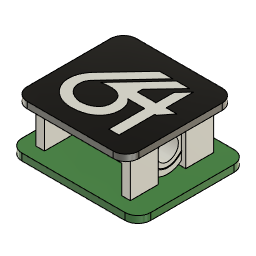
C64_logo_illuminated_multi v5 (Autodesk Fusion 360 design; units mm, degrees)
Autodesk Fusion 360 part; units mm, degrees
sketch "face plate" plane through (0, 0, 0) normal (0, 0, 1) x (1, 0, 0) in component "Face Plate"
  arc A0 (13, 9.7) -> (10, 12.7) centre (10, 9.7) ccw
  arc A1 (-13, -9.7) -> (-10, -12.7) centre (-10, -9.7) ccw
  arc A2 (10, -12.7) -> (13, -9.7) centre (10, -9.7) ccw
  line L0 (-13, 12.7) -> (13, -12.7) construction
  line L1 (-10, -12.7) -> (10, -12.7)
  arc A3 (-10, 12.7) -> (-13, 9.7) centre (-10, 9.7) ccw
  line L2 (10, 12.7) -> (-10, 12.7)
  line L3 (13, -9.7) -> (13, 9.7)
  line L4 (-10, 9.7) -> (10, -9.7) construction
  line L5 (13, 12.7) -> (-13, -12.7) construction
  line L6 (-10, -9.7) -> (10, -9.7) construction
  line L7 (10, 9.7) -> (-10, -9.7) construction
  line L8 (10, 9.7) -> (-10, 9.7) construction
  line L9 (-13, 9.7) -> (-13, -9.7)
  line L10 (10, -9.7) -> (10, 9.7) construction
  line L11 (-10, 9.7) -> (-10, -9.7) construction
  spline S0 degree 3 poles (2.5906, -3.5962) (2.5376, -1.7674) (1.7387, -0.8132) (1.1259, -0.4461) knots 0 0 0 0 1 1 1 1
  line L12 (2.5906, -3.5962) -> (2.5376, -1.7674)
  line L13 (2.5376, -1.7674) -> (1.7387, -0.8132)
  line L14 (1.7387, -0.8132) -> (1.1259, -0.4461)
  spline S1 degree 3 poles (-9.888, -3.2279) (-9.888, -6.2686) (-7.0983, -8.7953) (-3.8691, -8.7953) knots 0 0 0 0 1 1 1 1
  line L15 (-9.888, -3.2279) -> (-9.888, -6.2686)
  line L16 (-9.888, -6.2686) -> (-7.0983, -8.7953)
  line L17 (-7.0983, -8.7953) -> (-3.8691, -8.7953)
  line L18 (7.4492, -8.7953) -> (7.4492, -0.4461)
  line L19 (7.4492, -0.4461) -> (7.8267, -0.4474)
  spline S2 degree 3 poles (-3.8691, -8.7953) (0.9243, -8.7953) (2.6578, -5.9391) (2.5906, -3.5962) knots 0 0 0 0 1 1 1 1
  line L20 (-3.8691, -8.7953) -> (0.9243, -8.7953)
  line L21 (0.9243, -8.7953) -> (2.6578, -5.9391)
  line L22 (2.6578, -5.9391) -> (2.5906, -3.5962)
  spline S3 degree 3 poles (-3.8684, -6.5605) (-4.8205, -6.5605) (-7.4292, -5.7507) (-7.5798, -3.3049) knots 0 0 0 0 1 1 1 1
  line L23 (-3.8684, -6.5605) -> (-4.8205, -6.5605)
  line L24 (-4.8205, -6.5605) -> (-7.4292, -5.7507)
  line L25 (-7.4292, -5.7507) -> (-7.5798, -3.3049)
  line L26 (5.0693, -0.4461) -> (5.0693, -8.7953)
  line L27 (5.0693, -8.7953) -> (7.4492, -8.7953)
  spline S4 degree 2 poles (-7.5798, -3.3049) (-7.6755, -1.7654) (-6.5786, -0.7329) knots 0 0 0 1 1 1
  line L28 (-7.5798, -3.3049) -> (-7.6755, -1.7654)
  line L29 (-7.6755, -1.7654) -> (-6.5786, -0.7329)
  spline S5 degree 3 poles (0.1739, -3.0822) (0.2818, -5.6121) (-1.9966, -6.5605) (-3.8684, -6.5605) knots 0 0 0 0 1 1 1 1
  line L30 (0.1739, -3.0822) -> (0.2818, -5.6121)
  line L31 (0.2818, -5.6121) -> (-1.9966, -6.5605)
  line L32 (-1.9966, -6.5605) -> (-3.8684, -6.5605)
  line L33 (7.8267, -0.4474) -> (9.9138, 2.2094)
  spline S6 degree 2 poles (-5.295, -0.3005) (0.0123, 0.7243) (0.1739, -3.0822) knots 0 0 0 1 1 1
  line L34 (-5.295, -0.3005) -> (0.0123, 0.7243)
  line L35 (0.0123, 0.7243) -> (0.1739, -3.0822)
  line L36 (5.2394, 2.0437) -> (0.9553, 2.0437)
  spline S7 degree 2 poles (-8.3212, 0.7243) (-9.888, -1.1323) (-9.888, -3.2279) knots 0 0 0 1 1 1
  line L37 (-8.3212, 0.7243) -> (-9.888, -1.1323)
  line L38 (-9.888, -1.1323) -> (-9.888, -3.2279)
  line L39 (-0.6729, 8.8158) -> (-8.3212, 0.7243)
  line L40 (0.9553, 3.1785) -> (6.2962, 8.8158)
  line L41 (7.4493, 8.5608) -> (5.2394, 6.181)
  line L42 (-6.5786, -0.7329) -> (2.3527, 8.8159)
  line L43 (5.2394, 6.181) -> (5.2394, 2.0437)
  line L44 (7.4493, 2.2094) -> (7.4493, 8.5608)
  line L45 (6.2962, 8.8158) -> (3.237, 8.8158)
  line L46 (2.3527, 8.8159) -> (-0.6729, 8.8158)
  line L47 (1.1259, -0.4461) -> (5.0693, -0.4461)
  line L48 (3.237, 8.8158) -> (-5.295, -0.3005)
  line L49 (0.9553, 2.0437) -> (0.9553, 3.1785)
  line L50 (9.9138, 2.2094) -> (7.4493, 2.2094)
  dimension "d101" = 20
  dimension "d102" = 19.4
  dimension "d103" = 3
  dimension "d104" = 3
  dimension "d105" = 3
  dimension "d106" = 3
  dimension "d107" = 3
  dimension "d108" = 3
  constraint perpendicular L8 L11
  constraint parallel L6 L8
  constraint horizontal L8
  constraint parallel L1 L2
  constraint horizontal L2
  constraint coincident L5.end L9
  constraint coincident L5.end L1
  constraint tangent A1 L9
  constraint tangent A1 L1
  constraint coincident L0.end L1
  constraint coincident L0.end L3
  constraint tangent A2 L1
  constraint tangent A2 L3
  constraint coincident L5.start L2
  constraint coincident L5.start L3
  constraint tangent A0 L2
  constraint tangent A0 L3
  constraint coincident L0.start L9
  constraint coincident L0.start L2
  constraint tangent A3 L9
  constraint tangent A3 L2
  measures "d101" distance of A1.centre A2.centre
  measures "d102" distance of A3.centre A1.centre
  measures "d103" distance of L9 L11
  measures "d104" distance of L1 L6
  measures "d105" radius of A1
  measures "d106" radius of A2
  measures "d107" radius of A0
  measures "d108" radius of A3
sketch "illuminated body" plane through (0, 0, 0) normal (0, 0, 1) x (1, 0, 0) in component "Illuminated_Body_multi"
  line L0 (-10, 9.7) -> (-10, -9.7)
  line L1 (10, 9.7) -> (-10, 9.7)
  line L2 (10, -9.7) -> (10, 9.7)
  line L3 (-10, -9.7) -> (10, -9.7)
  spline S0 degree 3 poles (-9.888, -3.2279) (-9.888, -6.2686) (-7.0983, -8.7953) (-3.8691, -8.7953) knots 0 0 0 0 1 1 1 1
  spline S1 degree 2 poles (-8.3212, 0.7243) (-9.888, -1.1323) (-9.888, -3.2279) knots 0 0 0 1 1 1
  line L4 (-0.6729, 8.8158) -> (-8.3212, 0.7243)
  line L5 (2.3527, 8.8159) -> (-0.6729, 8.8158)
  line L6 (-6.5786, -0.7329) -> (2.3527, 8.8159)
  spline S2 degree 2 poles (-7.5798, -3.3049) (-7.6755, -1.7654) (-6.5786, -0.7329) knots 0 0 0 1 1 1
  spline S3 degree 3 poles (-3.8684, -6.5605) (-4.8205, -6.5605) (-7.4292, -5.7507) (-7.5798, -3.3049) knots 0 0 0 0 1 1 1 1
  spline S4 degree 3 poles (0.1739, -3.0822) (0.2818, -5.6121) (-1.9966, -6.5605) (-3.8684, -6.5605) knots 0 0 0 0 1 1 1 1
  spline S5 degree 2 poles (-5.295, -0.3005) (0.0123, 0.7243) (0.1739, -3.0822) knots 0 0 0 1 1 1
  line L7 (3.237, 8.8158) -> (-5.295, -0.3005)
  line L8 (6.2962, 8.8158) -> (3.237, 8.8158)
  line L9 (0.9553, 3.1785) -> (6.2962, 8.8158)
  line L10 (0.9553, 2.0437) -> (0.9553, 3.1785)
  line L11 (5.2394, 2.0437) -> (0.9553, 2.0437)
  line L12 (5.2394, 6.181) -> (5.2394, 2.0437)
  line L13 (7.4493, 8.5608) -> (5.2394, 6.181)
  line L14 (7.4493, 2.2094) -> (7.4493, 8.5608)
  line L15 (9.9138, 2.2094) -> (7.4493, 2.2094)
  line L16 (7.8267, -0.4474) -> (9.9138, 2.2094)
  line L17 (7.4492, -0.4461) -> (7.8267, -0.4474)
  line L18 (7.4492, -8.7953) -> (7.4492, -0.4461)
  line L19 (5.0693, -8.7953) -> (7.4492, -8.7953)
  line L20 (5.0693, -0.4461) -> (5.0693, -8.7953)
  line L21 (1.1259, -0.4461) -> (5.0693, -0.4461)
  spline S6 degree 3 poles (2.5906, -3.5962) (2.5376, -1.7674) (1.7387, -0.8132) (1.1259, -0.4461) knots 0 0 0 0 1 1 1 1
  spline S7 degree 3 poles (-3.8691, -8.7953) (0.9243, -8.7953) (2.6578, -5.9391) (2.5906, -3.5962) knots 0 0 0 0 1 1 1 1
extrude "Extrude1" add sketch "illuminated body" against normal blind 1 contours L0 L1 L2 L3 | S0 S1 L4 L5 L6 S2 S3 S4 S5 L7 L8 L9 L10 L11 L12 L13 L14 L15 L16 L17 L18 L19 L20 L21 S6 S7 makes body 1 in component "Illuminated_Body_multi"
extrude "Extrude2" add sketch "face plate" along normal blind 1.5 contours S0 S1 L18 L19 S2 L23 L24 L25 L26 L27 L28 L29 L30 L31 L32 L33 L34 L35 L36 S7 L39 L40 L41 L42 L43 L44 L45 L46 L47 L48 L49 L50 | S4 L28 L29 | S3 L23 L24 L25 | S5 L30 L31 L32 | S6 L34 L35 bodies 1 in component "Illuminated_Body_multi"
extrude "Extrude1'" add sketch "face plate" along normal blind 1.5 separate body contours A0 A1 A2 L1 A3 L2 L3 L9 | S0 L12 L13 L14 | S2 L20 L21 L22 | S1 L15 L16 L17 | S7 L37 L38 makes body 2 in component "Face Plate"
sketch "led insert" plane through (10, 0, 0) normal (1, 0, 0) x (0, 1, 0) in component "Illuminated_Body_multi"
  line L0 (9.7, 0) -> (-9.7, 0)
  line L1 (-9.7, 0) -> (-9.7, -1)
  line L2 (-9.7, -1) -> (9.7, -1)
  line L3 (9.7, -1) -> (9.7, 0)
  line L4 (0, -1) -> (0, -9.1868) construction
  line L5 (-9.7, -1) -> (-2.2348, -7.1936)
  line L6 (-9.7, -1) -> (9.7, -1)
  line L7 (9.7, -1) -> (2.2348, -7.1936)
  circle A0 centre (0, -4.5) radius 2.5
  line L8 (9.7, -1) -> (-9.7, -1)
  arc A1 (-2.2348, -7.1936) -> (2.2348, -7.1936) centre (0, -4.5) ccw
  dimension "d115" = 5
  dimension "d116" = 3.5
  dimension "d117" = 7
  constraint midpoint L4.start L6
  constraint coincident A0.centre L4
  constraint concentric A0 A1
  constraint coincident L1.end L2.start
  constraint tangent L5 A1
  constraint coincident L2.end L3.start
  constraint tangent L7 A1
  measures "d115" diameter of A0
  measures "d116" distance of A0.centre L8
  measures "d117" diameter of A1
extrude "Extrude3" add sketch "led insert" against normal blind 20 contours L2 L5 L6 L7 L8 A1 bodies 1 in component "Illuminated_Body_multi"
sketch "reflector" plane through (10, 0, 0) normal (1, 0, 0) x (0, 1, 0) in component "Refector"
  circle A0 centre (0, -4.5) radius 2.5
  line L0 (9.7, 0) -> (-9.7, 0)
  line L1 (-9.7, 0) -> (-9.7, -1)
  line L2 (-9.7, -1) -> (-2.2348, -7.1936)
  arc A1 (-2.2348, -7.1936) -> (2.2348, -7.1936) centre (0, -4.5) ccw
  line L3 (2.2348, -7.1936) -> (9.7, -1)
  line L4 (9.7, -1) -> (9.7, 0)
  line L5 (-9.7, -2.949) -> (-9.7, -9.5)
  line L6 (-3.2, -9.5) -> (-9.7, -9.5)
  line L7 (9.7, -1) -> (9.7, 0)
  line L8 (9.7, -1.2599) -> (9.7, -2.949)
  arc A2 (-3.1926, -8.348) -> (3.1926, -8.348) centre (0, -4.5) ccw
  line L9 (0, -9.5) -> (9.7, -9.5)
  arc A3 (-2.3625, -7.3475) -> (2.3625, -7.3475) centre (0, -4.5) ccw
  line L10 (9.7, -1.2599) -> (3.2, -1.2599)
  line L11 (3.1926, -8.348) -> (9.7, -2.949)
  line L12 (9.7, -9.5) -> (9.7, -2.949)
  line L13 (-9.7, 0) -> (-9.7, -1)
  line L14 (-9.7, -1.2599) -> (-9.7, -2.949)
  line L15 (3.2, -9.5) -> (9.7, -9.5)
  line L16 (-9.7, -1.2599) -> (-2.3625, -7.3475)
  line L17 (-9.7, -9.5) -> (0, -9.5)
  circle A4 centre (0, -4.5) radius 2.5
  line L18 (-3.2, -1.2599) -> (-3.2, -9.5)
  line L19 (-9.7, -2.949) -> (-3.1926, -8.348)
  line L20 (-9.7, -9.5) -> (-9.7, -1.2599)
  line L21 (-9.7, -1.2599) -> (-3.2, -1.2599)
  line L22 (3.2, -1.2599) -> (3.2, -9.5)
  line L23 (2.3625, -7.3475) -> (9.7, -1.2599)
  line L24 (9.7, 0) -> (-9.7, 0)
  line L25 (9.7, -9.5) -> (9.7, -1.2599)
  line L26 (-9.7, -1) -> (-2.2348, -7.1936) construction
  arc A5 (-2.2348, -7.1936) -> (2.2348, -7.1936) centre (0, -4.5) ccw construction
  line L27 (9.7, -1) -> (2.2348, -7.1936) construction
  line L28 (9.7, -1) -> (9.7, 0) construction
  line L29 (-9.7, 0) -> (9.7, 0) construction
  line L30 (-9.7, 0) -> (-9.7, -1) construction
  dimension "d121" = 1.3
  dimension "d122" = 9.7
  dimension "d123" = 19.4
  dimension "d124" = 6.5
  dimension "d125" = 6.5
  constraint tangent A2 L11
  constraint tangent A2 L19
  constraint tangent A3 L16
  constraint tangent A3 L23
  constraint vertical L14
  constraint parallel L8 L14
  constraint parallel L5 L14
  constraint midpoint L9.start A2
  constraint tangent A2 L17
  constraint tangent A2 L9
  constraint perpendicular L8 L9
  constraint perpendicular L9 L12
  constraint horizontal L21
  constraint vertical L18
  constraint horizontal L6
  constraint vertical L20
  constraint coincident L6.start L17
  constraint horizontal L10
  constraint vertical L22
  constraint horizontal L15
  constraint vertical L25
  constraint coincident L15.start L9
  measures "d121" distance of L16 L19
  measures "d122" horizontal distance of origin L14.start
  measures "d123" distance of L9.end L5.end
  measures "d124" distance of L5 L18
  measures "d125" distance of L12 L22
extrude "Extrude1''" add sketch "reflector" along normal blind 1 separate body contours L3 L10 L22 L23 | L3 L10 L22 | L2 L18 L21 | L2 L16 L18 L21 | L8 L11 L22 L23 L25 | L14 L16 L18 L19 L20 | L9 L11 L12 L15 L22 L25 | L5 L6 L17 L18 L19 L20 makes body 3 at (10, -7.5333, -4.0066) makes body 4 at (10, 5.3667, -6.7533) in component "Refector"
extrude "Extrude2'" add sketch "reflector" against normal blind 20 contours L8 L11 L22 L23 L25 | L14 L16 L18 L19 L20 | A2 A3 L11 L16 L18 L19 L22 L23 bodies 3 4 in component "Refector"
extrude "Extrude3'" add sketch "reflector" against normal blind 1 from surface at -20 contours L3 L10 L22 L23 | L3 L10 L22 | L2 L18 L21 | L2 L16 L18 L21 | L8 L11 L22 L23 L25 | L14 L16 L18 L19 L20 | L9 L11 L12 L15 L22 L25 | L5 L6 L17 L18 L19 L20 bodies 3 in component "Refector"
ref_plane "WorkPlane2" through (0, 0, -9.5) normal (0, 0, 1) x (1, 0, 0) in component "PCB_logo"
sketch "Sketch1" plane through (0, 0, -9.5) normal (0, 0, 1) x (1, 0, 0) in component "PCB_logo"
  line L0 (11, 9.7) -> (8.5, 9.7)
  line L1 (8.5, 9.7) -> (8.5, 0)
  line L2 (8.5, 0) -> (8.5, -9.7)
  line L3 (8.5, -9.7) -> (11, -9.7)
  line L4 (11, -9.7) -> (11, -3.2)
  line L5 (11, -3.2) -> (10, -3.2)
  line L6 (10, -3.2) -> (10, 3.2)
  line L7 (10, 3.2) -> (11, 3.2)
  line L8 (11, 3.2) -> (11, 9.7)
  line L9 (7.4544, -0.4024) -> (10.7744, -3.7224)
  line L10 (0.0244, -0.0224) -> (-3.8506, -0.0224)
  line L11 (3.4944, -0.4024) -> (7.4544, -0.4024)
  line L12 (10.7744, -9.7224) -> (10.7744, 9.6776)
  line L13 (10.7744, 3.6776) -> (7.4544, 0.3576)
  line L14 (3.4944, 0.3576) -> (7.4544, 0.3576)
  line L15 (10.7744, -3.7224) -> (3.4944, -3.7224)
  line L16 (3.4944, 3.6776) -> (3.4944, 0.3576)
  line L17 (10.7744, -3.7224) -> (3.4944, -3.7224)
  line L18 (3.4944, -0.4024) -> (7.4544, -0.4024)
  line L19 (3.4944, -4.3778) -> (3.4944, -9.2403)
  line L20 (-9.2256, 9.6776) -> (-9.2256, -9.7224)
  line L21 (3.4944, 3.6776) -> (10.7744, 3.6776)
  line L22 (-9.2256, -9.7224) -> (10.7744, -9.7224)
  line L23 (3.4944, 9.1955) -> (3.4944, 4.333)
  arc A0 (3.4944, 4.333) -> (3.4944, -4.3779) centre (0.4746, -0.0224) ccw
  line L24 (10.7744, 9.6776) -> (-9.2256, 9.6776)
  line L25 (10.7744, -0.0224) -> (6.8994, -0.0224)
  line L26 (3.4944, -4.3778) -> (3.4944, -9.2403)
  line L27 (3.4944, 9.1955) -> (3.4944, 4.333)
  line L28 (5.3994, -0.0224) -> (1.5244, -0.0224)
  line L29 (7.4544, 0.3576) -> (10.7744, 3.6776)
  arc A1 (3.4944, 4.333) -> (3.4944, -4.3779) centre (0.4746, -0.0224) ccw
  arc A2 (3.4944, 9.1954) -> (3.4944, -9.2403) centre (0.4744, -0.0224) ccw
  line L30 (7.4544, -0.4024) -> (10.7744, -3.7224)
  line L31 (-9.3681, 2.5176) -> (-9.3681, -2.5624)
  line L32 (-9.6856, 2.8351) -> (-9.6856, 1.4776)
  circle A3 centre (-11.6856, -5.1024) radius 0.9525
  line L33 (-11.2256, 1.4776) -> (-9.6856, 1.4776)
  line L34 (-11.2256, -0.9224) -> (-9.6856, -0.9224)
  line L35 (3.4944, -3.7224) -> (3.4944, -0.4024)
  circle A4 centre (-11.6856, -7.6424) radius 0.9525
  line L36 (3.4944, -3.7224) -> (3.4944, -0.4024)
  line L37 (-9.6856, 0.8776) -> (-9.6856, -0.9224)
  line L38 (3.4944, 0.3576) -> (3.4944, 3.6776)
  line L39 (10.7744, 3.6776) -> (3.4944, 3.6776)
  line L40 (7.4544, 0.3576) -> (3.4944, 0.3576)
  line L41 (-11.2256, 0.8776) -> (-9.6856, 0.8776)
  line L42 (-11.2256, -1.5224) -> (-9.6856, -1.5224)
  line L43 (-9.3681, 2.8351) -> (-9.6856, 2.8351)
  line L44 (10.7744, 3.6776) -> (7.4544, 0.3576)
  line L45 (-9.6856, -0.9224) -> (-9.6856, -1.5224)
  line L46 (-9.6856, -2.5624) -> (-9.3681, -2.5624)
  line L47 (-9.6856, 1.4776) -> (-9.6856, 0.8776)
  line L48 (-9.3681, 2.5176) -> (-9.3681, 2.8351)
  arc A5 (3.4944, 9.1954) -> (3.4944, -9.2403) centre (0.4744, -0.0224) ccw
  line L49 (-9.6856, -1.5224) -> (-9.6856, -2.5624)
  line L50 (-3.1943, 9.6426) -> (4.4257, 9.6426)
  line L51 (11.2344, 2.5176) -> (10.9169, 2.5176)
  line L52 (-3.1943, 12.1826) -> (-3.1943, 9.6426)
  line L53 (10.9169, -2.8799) -> (11.2344, -2.8799)
  line L54 (4.7469, -9.6424) -> (-2.8731, -9.6424)
  line L55 (-2.8731, -12.1824) -> (4.7469, -12.1824)
  line L56 (12.7744, -1.5224) -> (11.2344, -1.5224)
  line L57 (12.7744, 1.4776) -> (11.2344, 1.4776)
  line L58 (10.9169, -2.5624) -> (10.9169, -2.8799)
  line L59 (4.4257, 9.6426) -> (4.4257, 12.1826)
  line L60 (-2.8731, -9.6424) -> (-2.8731, -12.1824)
  line L61 (12.7744, -0.9224) -> (11.2344, -0.9224)
  line L62 (4.4257, 10.9126) -> (5.1877, 10.9126)
  line L63 (12.7744, 0.8776) -> (11.2344, 0.8776)
  line L64 (11.2344, 0.8776) -> (11.2344, 1.4776)
  line L65 (4.4257, 12.1826) -> (-3.1943, 12.1826)
  line L66 (11.2344, 1.4776) -> (11.2344, 2.5176)
  line L67 (11.2344, -1.5224) -> (11.2344, -0.9224)
  line L68 (10.9169, -2.5624) -> (10.9169, 2.5176)
  line L69 (11.2344, -2.8799) -> (11.2344, -1.5224)
  line L70 (7.4243, -1.1337) -> (7.4274, -1.1337)
  line L71 (4.7469, -10.9124) -> (5.5089, -10.9124)
  line L72 (4.7469, -12.1824) -> (4.7469, -9.6424)
  line L73 (-2.8731, -10.9124) -> (-3.6351, -10.9124)
  line L74 (-3.1943, 10.9126) -> (-3.9563, 10.9126)
  line L75 (11.2344, -0.9224) -> (11.2344, 0.8776)
  arc A6 (-11.2256, 12.6776) -> (-14.2256, 9.6776) centre (-11.2256, 9.6776) ccw
  line L76 (12.7744, -12.7224) -> (-11.2256, -12.7224)
  line L77 (15.7744, 9.6776) -> (15.7744, -9.7224)
  line L78 (-11.2256, 12.6776) -> (12.7744, 12.6776)
  line L79 (-14.2256, -9.7224) -> (-14.2256, 9.6776)
  arc A7 (-14.2256, -9.7224) -> (-11.2256, -12.7224) centre (-11.2256, -9.7224) ccw
  arc A8 (12.7744, -12.7224) -> (15.7744, -9.7224) centre (12.7744, -9.7224) ccw
  arc A9 (15.7744, 9.6776) -> (12.7744, 12.6776) centre (12.7744, 9.6776) ccw
  line L80 (-12.4256, 0.8776) -> (-11.2256, 0.8776)
  line L81 (-11.9396, -5.3564) -> (-11.4316, -5.3564)
  line L82 (-11.9396, -4.8484) -> (-11.9396, -5.3564)
  line L83 (-11.2256, -0.9224) -> (-12.4256, -0.9224)
  line L84 (13.8744, 1.4776) -> (12.7744, 1.4776)
  line L85 (13.9744, 1.4776) -> (13.8744, 1.4776)
  line L86 (13.9744, -0.9224) -> (12.7744, -0.9224)
  line L87 (13.9744, 0.8776) -> (13.9744, 1.4776)
  line L88 (12.7744, 0.8776) -> (13.9744, 0.8776)
  line L89 (-11.2256, 1.4776) -> (-12.4256, 1.4776)
  line L90 (-11.4316, -5.3564) -> (-11.4316, -4.8484)
  line L91 (-11.4316, -7.3884) -> (-11.9396, -7.3884)
  line L92 (-12.4256, -1.5224) -> (-12.3256, -1.5224)
  line L93 (-12.3256, -1.5224) -> (-11.2256, -1.5224)
  line L94 (13.9744, -1.5224) -> (13.9744, -0.9224)
  line L95 (-11.4316, -7.8964) -> (-11.4316, -7.3884)
  line L96 (-11.9396, -7.3884) -> (-11.9396, -7.8964)
  line L97 (-11.9396, -7.8964) -> (-11.4316, -7.8964)
  line L98 (-12.4256, 1.4776) -> (-12.4256, 0.8776)
  line L99 (-12.4256, -0.9224) -> (-12.4256, -1.5224)
  line L100 (-11.4316, -4.8484) -> (-11.9396, -4.8484)
  line L101 (12.7744, -1.5224) -> (13.9744, -1.5224)
extrude "Extrude1'''" add sketch "Sketch1" against normal blind 1.6 separate body contours L0 L1 L7 L8 L12 L24 | L1 L12 L21 L24 L39 | L1 L2 L3 L9 L11 L12 L13 L14 L15 L16 L17 L18 L19 L21 L22 L23 A0 L24 L26 L27 L29 A1 A2 L30 L35 L36 L38 L39 L40 L44 A5 L50 L54 L59 L72 | L6 L7 L12 L13 L25 L29 L44 | L7 L12 L13 L29 L44 | L1 L6 L7 L13 L21 L29 L39 L44 | L1 L13 L14 L16 L21 L29 L38 L39 L40 L44 | L24 A2 A5 L50 L59 | L24 L52 L59 L65 | L6 L7 L13 L29 L44 | L5 L6 L9 L12 L25 L30 | L1 L2 L6 L13 L25 L29 L44 | L24 A2 A5 L50 L52 | A2 A5 L50 | L5 L9 L12 L30 | L3 L4 L5 L12 | L2 L6 L9 L25 L30 | L20 L24 A2 A5 L50 L52 | L19 L23 A0 L26 L27 A1 A2 A5 L50 L54 | L2 L5 L6 L9 L15 L17 L30 | L5 L6 L9 L30 | L2 L3 L12 L15 L17 | L20 L22 A2 A5 L54 L60 | L2 L9 L11 L15 L17 L18 L30 L35 L36 | A2 A5 L54 | L22 A2 A5 L54 L60 | L22 L55 L60 L72 | L22 A2 A5 L54 L72 | L31 L32 L37 L43 L45 L46 L47 L48 L49 | L34 L42 L45 L83 L92 L93 L99 | L33 L41 L47 L80 L89 L98 | A3 | A4 | L51 L53 L58 L64 L66 L67 L68 L69 L75 | L57 L63 L64 L84 L85 L87 L88 | L56 L61 L67 L86 L94 L101 | A6 L76 L77 L78 L79 A7 A8 A9 | L81 L82 L90 L100 | L91 L95 L96 L97 makes body 5 in component "PCB_logo"
extrude "Extrude2''" cut sketch "Sketch1" against normal blind 1.6 contours L81 L82 L90 L100 | L91 L95 L96 L97 bodies 5 in component "PCB_logo"
sketch "Sketch10" plane through (0, 0, 0) normal (0, 0, 1) x (1, 0, 0)
  line L0 (-0.6729, 8.8158) -> (-8.3212, 0.7243)
  spline S0 degree 2 poles (-8.3212, 0.7243) (-9.888, -1.1323) (-9.888, -3.2279) knots 0 0 0 1 1 1
  line L1 (-8.3212, 0.7243) -> (-9.888, -1.1323)
  line L2 (-9.888, -1.1323) -> (-9.888, -3.2279)
  spline S1 degree 3 poles (-9.888, -3.2279) (-9.888, -6.2686) (-7.0983, -8.7953) (-3.8691, -8.7953) knots 0 0 0 0 1 1 1 1
  line L3 (-9.888, -3.2279) -> (-9.888, -6.2686)
  line L4 (-9.888, -6.2686) -> (-7.0983, -8.7953)
  line L5 (-7.0983, -8.7953) -> (-3.8691, -8.7953)
  spline S2 degree 3 poles (-3.8691, -8.7953) (0.9243, -8.7953) (2.6578, -5.9391) (2.5906, -3.5962) knots 0 0 0 0 1 1 1 1
  line L6 (-3.8691, -8.7953) -> (0.9243, -8.7953)
  line L7 (0.9243, -8.7953) -> (2.6578, -5.9391)
  line L8 (2.6578, -5.9391) -> (2.5906, -3.5962)
  spline S3 degree 3 poles (2.5906, -3.5962) (2.5376, -1.7674) (1.7387, -0.8132) (1.1259, -0.4461) knots 0 0 0 0 1 1 1 1
  line L9 (2.5906, -3.5962) -> (2.5376, -1.7674)
  line L10 (2.5376, -1.7674) -> (1.7387, -0.8132)
  line L11 (1.7387, -0.8132) -> (1.1259, -0.4461)
  line L12 (1.1259, -0.4461) -> (5.0693, -0.4461)
  line L13 (5.0693, -0.4461) -> (5.0693, -8.7953)
  line L14 (5.0693, -8.7953) -> (7.4492, -8.7953)
  line L15 (7.4492, -8.7953) -> (7.4492, -0.4461)
  line L16 (7.4492, -0.4461) -> (7.8267, -0.4474)
  line L17 (7.8267, -0.4474) -> (9.9138, 2.2094)
  line L18 (9.9138, 2.2094) -> (7.4493, 2.2094)
  line L19 (7.4493, 2.2094) -> (7.4493, 8.5608)
  line L20 (7.4493, 8.5608) -> (5.2394, 6.181)
  line L21 (5.2394, 6.181) -> (5.2394, 2.0437)
  line L22 (5.2394, 2.0437) -> (0.9553, 2.0437)
  line L23 (0.9553, 2.0437) -> (0.9553, 3.1785)
  line L24 (0.9553, 3.1785) -> (6.2962, 8.8158)
  line L25 (6.2962, 8.8158) -> (3.237, 8.8158)
  line L26 (3.237, 8.8158) -> (-5.295, -0.3005)
  spline S4 degree 2 poles (-5.295, -0.3005) (0.0123, 0.7243) (0.1739, -3.0822) knots 0 0 0 1 1 1
  line L27 (-5.295, -0.3005) -> (0.0123, 0.7243)
  line L28 (0.0123, 0.7243) -> (0.1739, -3.0822)
  spline S5 degree 3 poles (0.1739, -3.0822) (0.2818, -5.6121) (-1.9966, -6.5605) (-3.8684, -6.5605) knots 0 0 0 0 1 1 1 1
  line L29 (0.1739, -3.0822) -> (0.2818, -5.6121)
  line L30 (0.2818, -5.6121) -> (-1.9966, -6.5605)
  line L31 (-1.9966, -6.5605) -> (-3.8684, -6.5605)
  spline S6 degree 3 poles (-3.8684, -6.5605) (-4.8205, -6.5605) (-7.4292, -5.7507) (-7.5798, -3.3049) knots 0 0 0 0 1 1 1 1
  line L32 (-3.8684, -6.5605) -> (-4.8205, -6.5605)
  line L33 (-4.8205, -6.5605) -> (-7.4292, -5.7507)
  line L34 (-7.4292, -5.7507) -> (-7.5798, -3.3049)
  spline S7 degree 2 poles (-7.5798, -3.3049) (-7.6755, -1.7654) (-6.5786, -0.7329) knots 0 0 0 1 1 1
  line L35 (-7.5798, -3.3049) -> (-7.6755, -1.7654)
  line L36 (-7.6755, -1.7654) -> (-6.5786, -0.7329)
  line L37 (-6.5786, -0.7329) -> (2.3527, 8.8159)
  line L38 (2.3527, 8.8159) -> (-0.6729, 8.8158)
  line L39 (-9.9606, 10.0103) -> (10.0394, 10.0103)
  line L40 (10.0394, 10.0103) -> (10.0394, -9.9897)
  line L41 (10.0394, -9.9897) -> (-9.9606, -9.9897)
  line L42 (-9.9606, -9.9897) -> (-9.9606, 10.0103)
extrude "Extrude4" add 2 faces at (-10, -7.5333, -6.9303) (-10, 7.5333, -6.9303) along direction (1, 0, 0) blind 1 on bodies 3 bodies 3 in component "Refector"
extrude "Extrude5" add 2 faces at (10, -7.5333, -6.9303) (10, 7.5333, -6.9303) along direction (-1, 0, 0) blind 1 on bodies 3 bodies 3 in component "Refector"
component "Face Plate" placed x (1, 0, 0) y (0, 1, 0) z (0, 0, 1) at (0, 0, 0)
component "Illuminated_Body_multi" placed x (1, 0, 0) y (0, 1, 0) z (0, 0, 1) at (0, 0, 0)
component "Refector" placed x (1, 0, 0) y (0, 1, 0) z (0, 0, 1) at (0, 0, 0)
component "PCB_logo" placed x (1, 0, 0) y (0, 1, 0) z (0, 0, 1) at (0, 0, 0)
equation "baselineA = 20 mm"
equation "framedistance = 3 mm"
equation "height_logo = 5 mm"
equation "height_baseplate = 1.5 mm"
equation "height_below = 2 mm"
equation "distance_baseplate = 0.0 mm"
equation "d101 = baselineA"
equation "d102 = baselineA * 0.97"
equation "d103 = framedistance"
equation "d104 = framedistance"
equation "d105 = framedistance"
equation "d106 = framedistance"
equation "d107 = framedistance"
equation "d108 = framedistance"
equation "d111 = height_baseplate"
equation "d113 = height_baseplate"
named bodies: "pcb_logo", "illuminated body", "face pate", "reflector"
